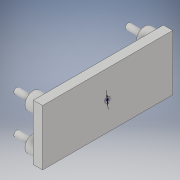
# Autodesk Inventor part: Part10
Saved by Autodesk Inventor 2019 (Build 230136000, 136)
## iProperties
Created: 2021-08-30
Part Number: Part10
Material: 一般
Document SubType Name: Sheet Metal
Designer: yuta
Density: 1 g/cm^3
Sheet Metal Rule: Default_mm
Appearance: 既定
Author: yuta
Autodesk Inventor part; units mm, degrees
ref_plane "YZ Plane" through (0, 0, 0) normal (1, 0, 0) x (0, 1, 0)
ref_plane "XZ Plane" through (0, 0, 0) normal (0, 1, 0) x (-1, 0, 0)
ref_plane "XY Plane" through (0, 0, 0) normal (0, 0, 1) x (1, 0, 0)
sketch "スケッチ1" plane through (0, 0, 0) normal (1, 0, 0) x (0, 1, 0)
  point P0 (0, 0)
sketch "スケッチ2" plane through (0, 0, 0) normal (1, 0, 0) x (0, 1, 0)
  line L0 (29.4185, 69.6387) -> (-30.5815, 69.6387)
  line L1 (-30.5815, 69.6387) -> (-30.5815, -70.3613)
  line L2 (-30.5815, -70.3613) -> (29.4185, -70.3613)
  line L3 (29.4185, -70.3613) -> (29.4185, 69.6387)
  point P0 (0, 0)
  dimension "d0" = 60
  dimension "d1" = 140
  constraints: 8 end point, 2 parallel, 1 horizontal, 1 perpendicular
  measures "d0" distance of L2.end L1.end
  measures "d1" distance of L1.end L0.end
extrude "押し出し1" add sketch "スケッチ2" along normal blind 10
sketch "スケッチ3" plane through (0, 0, 0) normal (-1, 0, 0) x (0, 0, 1)
  circle A0 centre (-60.3613, 19.4185) radius 9
  line L0 (-70.3613, 29.4185) -> (69.6387, 29.4185) projected
  line L1 (-70.3613, -30.5815) -> (-70.3613, 29.4185) projected
  circle A1 centre (-60.3613, -20.5815) radius 9
  line L2 (69.6387, -30.5815) -> (-70.3613, -30.5815) projected
  circle A2 centre (59.6387, -20.5815) radius 9
  line L3 (69.6387, 29.4185) -> (69.6387, -30.5815) projected
  circle A3 centre (59.6387, 19.4185) radius 9
  circle A4 centre (-60.3613, 19.4185) radius 8
  circle A5 centre (-60.3613, -20.5815) radius 8
  circle A6 centre (59.6387, 19.4185) radius 8
  circle A7 centre (59.6387, -20.5815) radius 8
  point P0 (0, 0)
  dimension "d4" = 18
  dimension "d5" = 10
  dimension "d6" = 10
  dimension "d7" = 18
  dimension "d8" = 10
  dimension "d9" = 18
  dimension "d10" = 10
  dimension "d11" = 18
  dimension "d12" = 16
  dimension "d13" = 16
  dimension "d14" = 16
  dimension "d15" = 16
  constraints: 8 centre point, 4 coincident
  measures "d4" diameter of A0
  measures "d5" distance from line of A0.centre L0
  measures "d6" distance from line of L1 A0.centre
  measures "d7" diameter of A1
  measures "d8" distance from line of L2 A1.centre
  measures "d9" diameter of A2
  measures "d10" distance from line of L3 A2.centre
  measures "d11" diameter of A3
  measures "d12" diameter of A4
  measures "d13" diameter of A5
  measures "d14" diameter of A6
  measures "d15" diameter of A7
extrude "押し出し2" add sketch "スケッチ3" along normal blind 10 contours A0 | A1 | A2 | A3
sketch "スケッチ4" plane through (0, 0, 0) normal (-1, 0, 0) x (0, 0, 1)
  point P0 (0, 0)
sketch "スケッチ5" plane through (0, 0, 0) normal (-1, 0, 0) x (0, 0, 1)
  circle A0 centre (-60.3613, 19.4185) radius 3
  line L0 (-70.3613, 29.4185) -> (69.6387, 29.4185) projected
  line L1 (-70.3613, -30.5815) -> (-70.3613, 29.4185) projected
  circle A1 centre (-60.3613, -20.5815) radius 3
  line L2 (69.6387, -30.5815) -> (-70.3613, -30.5815) projected
  circle A2 centre (59.6387, 19.4185) radius 3
  line L3 (69.6387, 29.4185) -> (69.6387, -30.5815) projected
  point P0 (0, 0)
  dimension "d18" = 6
  dimension "d19" = 10
  dimension "d20" = 10
  dimension "d21" = 6
  dimension "d22" = 10
  dimension "d23" = 6
  dimension "d24" = 10
  constraints: 3 centre point
  measures "d18" diameter of A0
  measures "d19" distance from line of L0 A0.centre
  measures "d20" distance from line of L1 A0.centre
  measures "d21" diameter of A1
  measures "d22" distance from line of L2 A1.centre
  measures "d23" diameter of A2
  measures "d24" distance from line of L3 A2.centre
sketch "スケッチ6" plane through (0, 0, 0) normal (-1, 0, 0) x (0, 0, 1)
  circle A0 centre (-60.3613, 19.4185) radius 3
  circle A1 centre (59.6387, 19.4185) radius 3
  circle A2 centre (59.6387, -20.5815) radius 3
  line L0 (69.6387, 29.4185) -> (69.6387, -30.5815) projected
  line L1 (69.6387, -30.5815) -> (-70.3613, -30.5815) projected
  point P0 (0, 0)
  dimension "d25" = 6
  dimension "d26" = 6
  dimension "d27" = 6
  dimension "d28" = 10
  dimension "d29" = 10
  constraints: 3 centre point
  measures "d25" diameter of A0
  measures "d26" diameter of A1
  measures "d27" diameter of A2
  measures "d28" distance from line of L0 A2.centre
  measures "d29" distance from line of L1 A2.centre
extrude "押し出し3" add sketch "スケッチ6" along normal blind 28
extrude "押し出し4" add sketch "スケッチ5" along normal blind 28 contours A1
sketch "スケッチ7" plane through (10, 0, 0) normal (1, 0, 0) x (0, 0, -1)
  point P0 (0, 0)
sketch "スケッチ8" plane through (10, 0, 0) normal (1, 0, 0) x (0, 0, -1)
  circle A0 centre (0, 0) radius 1
  dimension "d35" = 2
  constraints: 1 centre point, 1 coincident
  measures "d35" diameter of A0
sketch "スケッチ9" plane through (10, 0, 0) normal (1, 0, 0) x (0, 0, -1)
  circle A0 centre (0, 0) radius 3
  dimension "d36" = 6
  constraints: 1 centre point, 1 coincident
  measures "d36" diameter of A0
hole "穴1" at (10, 0, 0) direction (-1, 0, 0) diameter 6 depth 10
equation "\"BendRadius\" = Thickness"
equation "\"BendReliefWidth\" = Thickness"
equation "\"BendReliefDepth\" = 0.5 * Thickness"
equation "\"CornerReliefSize\" = 4 * Thickness"
equation "\"MinimumRemnant\" = 2 * Thickness"
equation "\"TransitionRadius\" = BendRadius"
equation "\"JacobiRadiusSize\" = BendRadius"
equation "\"GapSize\" = Thickness"
equation "\"Thickness\" = 0.5"
